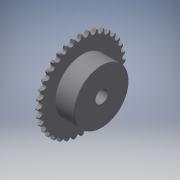
# Autodesk Inventor part: 22252-10380732036
Saved by Autodesk Inventor 2018 (Build 220112000, 112)
## iProperties
Category: PARTsolutions
Company: NORELEM
Created: 2018-08-05
Part Number: 22252-10380732036
Material: Generic
Catalog Web Link: www.cadenas.de
Description: 22252-Sprockets single 3/8“ x 7/32“ DIN ISO 606
Vendor: NORELEM
Document SubType Name: Modeling
Designer: psadmin
Manufacturer: NORELEM
Mass: 136.264 g
Surface Area: 270.64 cm^2
Volume: 136.264 cm^3
Density: 1 g/cm^3
Appearance: PSOLRGB-175-175-175
PSOL_IDENT_0: {$CADENAS_DATA\23d-libs\norelem\data\22000\22252.prj},174 {VTYP=3D},{NB=22252-10380732036},{LINA=222
PSOL_IDENT_1: 52-10380732036},{NN=22252},{DATE=25.07.2018 05:07:11},{GEOMDATE=17.06.2016 07:26:47},{VERSION=},{LIN
PSOL_IDENT_2: EID=430},{WBVAR=},{WBNUMERIC=}  {NB=22252-10380732036},{LINA=22252-10380732036},{KT=DUMMY},{BEST=222
PSOL_IDENT_3: 52-10380732036},{ISONR=06 B-1},{TZOLL=3/8\" x 7/32\"},{TMM=9,525 x 5,72},{ZZ=36},{D=113.0},{D1=109.2
PSOL_IDENT_4: 9},{D2=70},{D3=16},{B1=5.3},{L=30},{C=1},{R=10},{BS=Infotext},{INFO=Info},{FILTER=NORELEM,},{SAP=212
PSOL_IDENT_5: 278},{XC=1.300},{XD=6.350},{XF=1.800},{XG=0.000},{XH=0.000},{XI=0.000},{XJ=0.000},{XK=0.000},{XL=0.0
PSOL_IDENT_6: 00},{XM=0.000},{XN=0.000}
NN: 22252
NT: Sprockets single 3/8“ x 7/32“ DIN ISO 606
NB: 22252-10380732036
NBSYN: $BEST.
LINA: 22252-10380732036
BEST: 22252-10380732036
ISONR: 06 B-1
TZOLL: 3/8" x 7/32"
TMM: 9,525 x 5,72
ZZ: 36
D: 113
D1: 109.29
D2: 70
D3: 16
B1: 5.3
L: 30
C: 1
R: 10
BS: Infotext
INFO: Info
SUPPLIER: NORELEM
ARTICLENO: 22252-10380732036
BOMINFO: 22252-10380732036
CREATOR: CADENAS GmbH
Title: 22252-10380732036
Author: Cadenas PARTsolutions
Comments: Sprockets single 3/8“ x 7/32“ DIN ISO 606
Autodesk Inventor part; units mm, degrees
ref_plane "YZ Plane" through (0, 0, 0) normal (1, 0, 0) x (0, 1, 0)
ref_plane "XZ Plane" through (0, 0, 0) normal (0, 1, 0) x (-1, 0, 0)
ref_plane "XY Plane" through (0, 0, 0) normal (0, 0, 1) x (1, 0, 0)
sketch "Sketch_3" plane through (0, 0, 0) normal (1, 0, 0) x (0, 1, 0)
  arc A0 (0, 56.5) -> (-0.65, 56.4963) centre (0, 0) ccw
  line L0 (-0.65, 56.4963) -> (-1.7617, 53.3699)
  arc A1 (-4.485, 51.2642) -> (-1.7617, 53.3699) centre (-4.7626, 54.4371) ccw
  arc A2 (-7.5326, 52.8651) -> (-4.485, 51.2642) centre (-4.7626, 54.4371) ccw
  line L1 (-7.5326, 52.8651) -> (-9.1703, 55.7508)
  arc A3 (-9.1703, 55.7508) -> (-9.8111, 55.6416) centre (0, 0) ccw
  arc A4 (-9.8111, 55.6416) -> (-10.4506, 55.5251) centre (0, 0) ccw
  line L2 (-10.4506, 55.5251) -> (-11.0025, 52.2532)
  arc A5 (-13.3188, 49.7065) -> (-11.0025, 52.2532) centre (-14.1432, 52.783) ccw
  arc A6 (-16.5981, 50.7539) -> (-13.3188, 49.7065) centre (-14.1432, 52.783) ccw
  line L3 (-16.5981, 50.7539) -> (-18.7121, 53.3114)
  arc A7 (-18.7121, 53.3114) -> (-19.3241, 53.0926) centre (0, 0) ccw
  arc A8 (-19.3241, 53.0926) -> (-19.9337, 52.8668) centre (0, 0) ccw
  line L4 (-19.9337, 52.8668) -> (-19.9091, 49.5488)
  arc A9 (-21.7479, 46.6386) -> (-19.9091, 49.5488) centre (-23.094, 49.5252) ccw
  arc A10 (-25.1593, 47.1006) -> (-21.7479, 46.6386) centre (-23.094, 49.5252) ccw
  line L5 (-25.1593, 47.1006) -> (-27.6852, 49.2522)
  arc A11 (-27.6852, 49.2522) -> (-28.25, 48.9304) centre (0, 0) ccw
  arc A12 (-28.25, 48.9304) -> (-28.811, 48.6022) centre (0, 0) ccw
  line L6 (-28.811, 48.6022) -> (-28.2107, 45.3389)
  arc A13 (-29.5162, 42.1536) -> (-28.2107, 45.3389) centre (-31.3431, 44.7626) ccw
  arc A14 (-32.956, 42.0162) -> (-29.5162, 42.1536) centre (-31.3431, 44.7626) ccw
  line L7 (-32.956, 42.0162) -> (-35.8172, 43.6965)
  arc A15 (-35.8172, 43.6965) -> (-36.3175, 43.2815) centre (0, 0) ccw
  arc A16 (-36.3175, 43.2815) -> (-36.813, 42.8608) centre (0, 0) ccw
  line L8 (-36.813, 42.8608) -> (-35.6551, 39.7513)
  arc A17 (-36.3877, 36.3877) -> (-35.6551, 39.7513) centre (-38.6399, 38.6399) ccw
  arc A18 (-39.7513, 35.6551) -> (-36.3877, 36.3877) centre (-38.6399, 38.6399) ccw
  line L9 (-39.7513, 35.6551) -> (-42.8608, 36.813)
  arc A19 (-42.8608, 36.813) -> (-43.2815, 36.3175) centre (0, 0) ccw
  arc A20 (-43.2815, 36.3175) -> (-43.6965, 35.8172) centre (0, 0) ccw
  line L10 (-43.6965, 35.8172) -> (-42.0162, 32.956)
  arc A21 (-42.1536, 29.5162) -> (-42.0162, 32.956) centre (-44.7626, 31.3431) ccw
  arc A22 (-45.3389, 28.2107) -> (-42.1536, 29.5162) centre (-44.7626, 31.3431) ccw
  line L11 (-45.3389, 28.2107) -> (-48.6022, 28.811)
  arc A23 (-48.6022, 28.811) -> (-48.9304, 28.25) centre (0, 0) ccw
  arc A24 (-48.9304, 28.25) -> (-49.2522, 27.6852) centre (0, 0) ccw
  line L12 (-49.2522, 27.6852) -> (-47.1006, 25.1593)
  arc A25 (-46.6386, 21.7479) -> (-47.1006, 25.1593) centre (-49.5252, 23.094) ccw
  arc A26 (-49.5488, 19.9091) -> (-46.6386, 21.7479) centre (-49.5252, 23.094) ccw
  line L13 (-49.5488, 19.9091) -> (-52.8668, 19.9337)
  arc A27 (-52.8668, 19.9337) -> (-53.0926, 19.3241) centre (0, 0) ccw
  arc A28 (-53.0926, 19.3241) -> (-53.3114, 18.7121) centre (0, 0) ccw
  line L14 (-53.3114, 18.7121) -> (-50.7539, 16.5981)
  arc A29 (-49.7065, 13.3188) -> (-50.7539, 16.5981) centre (-52.783, 14.1432) ccw
  arc A30 (-52.2532, 11.0025) -> (-49.7065, 13.3188) centre (-52.783, 14.1432) ccw
  line L15 (-52.2532, 11.0025) -> (-55.5251, 10.4506)
  arc A31 (-55.5251, 10.4506) -> (-55.6416, 9.8111) centre (0, 0) ccw
  arc A32 (-55.6416, 9.8111) -> (-55.7508, 9.1703) centre (0, 0) ccw
  line L16 (-55.7508, 9.1703) -> (-52.8651, 7.5326)
  arc A33 (-51.2642, 4.485) -> (-52.8651, 7.5326) centre (-54.4371, 4.7626) ccw
  arc A34 (-53.3699, 1.7617) -> (-51.2642, 4.485) centre (-54.4371, 4.7626) ccw
  line L17 (-53.3699, 1.7617) -> (-56.4963, 0.65)
  arc A35 (-56.4963, 0.65) -> (-56.5, 0) centre (0, 0) ccw
  arc A36 (-56.5, 0) -> (-56.4963, -0.65) centre (0, 0) ccw
  line L18 (-56.4963, -0.65) -> (-53.3699, -1.7617)
  arc A37 (-51.2642, -4.485) -> (-53.3699, -1.7617) centre (-54.4371, -4.7626) ccw
  arc A38 (-52.8651, -7.5326) -> (-51.2642, -4.485) centre (-54.4371, -4.7626) ccw
  line L19 (-52.8651, -7.5326) -> (-55.7508, -9.1703)
  arc A39 (-55.7508, -9.1703) -> (-55.6416, -9.8111) centre (0, 0) ccw
  arc A40 (-55.6416, -9.8111) -> (-55.5251, -10.4506) centre (0, 0) ccw
  line L20 (-55.5251, -10.4506) -> (-52.2532, -11.0025)
  arc A41 (-49.7065, -13.3188) -> (-52.2532, -11.0025) centre (-52.783, -14.1432) ccw
  arc A42 (-50.7539, -16.5981) -> (-49.7065, -13.3188) centre (-52.783, -14.1432) ccw
  line L21 (-50.7539, -16.5981) -> (-53.3114, -18.7121)
  arc A43 (-53.3114, -18.7121) -> (-53.0926, -19.3241) centre (0, 0) ccw
  arc A44 (-53.0926, -19.3241) -> (-52.8668, -19.9337) centre (0, 0) ccw
  line L22 (-52.8668, -19.9337) -> (-49.5488, -19.9091)
  arc A45 (-46.6386, -21.7479) -> (-49.5488, -19.9091) centre (-49.5252, -23.094) ccw
  arc A46 (-47.1006, -25.1593) -> (-46.6386, -21.7479) centre (-49.5252, -23.094) ccw
  line L23 (-47.1006, -25.1593) -> (-49.2522, -27.6852)
  arc A47 (-49.2522, -27.6852) -> (-48.9304, -28.25) centre (0, 0) ccw
  arc A48 (-48.9304, -28.25) -> (-48.6022, -28.811) centre (0, 0) ccw
  line L24 (-48.6022, -28.811) -> (-45.3389, -28.2107)
  arc A49 (-42.1536, -29.5162) -> (-45.3389, -28.2107) centre (-44.7626, -31.3431) ccw
  arc A50 (-42.0162, -32.956) -> (-42.1536, -29.5162) centre (-44.7626, -31.3431) ccw
  line L25 (-42.0162, -32.956) -> (-43.6965, -35.8172)
  arc A51 (-43.6965, -35.8172) -> (-43.2815, -36.3175) centre (0, 0) ccw
  arc A52 (-43.2815, -36.3175) -> (-42.8608, -36.813) centre (0, 0) ccw
  line L26 (-42.8608, -36.813) -> (-39.7513, -35.6551)
  arc A53 (-36.3877, -36.3877) -> (-39.7513, -35.6551) centre (-38.6399, -38.6399) ccw
  arc A54 (-35.6551, -39.7513) -> (-36.3877, -36.3877) centre (-38.6399, -38.6399) ccw
  line L27 (-35.6551, -39.7513) -> (-36.813, -42.8608)
  arc A55 (-36.813, -42.8608) -> (-36.3175, -43.2815) centre (0, 0) ccw
  arc A56 (-36.3175, -43.2815) -> (-35.8172, -43.6965) centre (0, 0) ccw
  line L28 (-35.8172, -43.6965) -> (-32.956, -42.0162)
  arc A57 (-29.5162, -42.1536) -> (-32.956, -42.0162) centre (-31.3431, -44.7626) ccw
  arc A58 (-28.2107, -45.3389) -> (-29.5162, -42.1536) centre (-31.3431, -44.7626) ccw
  line L29 (-28.2107, -45.3389) -> (-28.811, -48.6022)
  arc A59 (-28.811, -48.6022) -> (-28.25, -48.9304) centre (0, 0) ccw
  arc A60 (-28.25, -48.9304) -> (-27.6852, -49.2522) centre (0, 0) ccw
  line L30 (-27.6852, -49.2522) -> (-25.1593, -47.1006)
  arc A61 (-21.7479, -46.6386) -> (-25.1593, -47.1006) centre (-23.094, -49.5252) ccw
  arc A62 (-19.9091, -49.5488) -> (-21.7479, -46.6386) centre (-23.094, -49.5252) ccw
  line L31 (-19.9091, -49.5488) -> (-19.9337, -52.8668)
  arc A63 (-19.9337, -52.8668) -> (-19.3241, -53.0926) centre (0, 0) ccw
  arc A64 (-19.3241, -53.0926) -> (-18.7121, -53.3114) centre (0, 0) ccw
  line L32 (-18.7121, -53.3114) -> (-16.5981, -50.7539)
  arc A65 (-13.3188, -49.7065) -> (-16.5981, -50.7539) centre (-14.1432, -52.783) ccw
  arc A66 (-11.0025, -52.2532) -> (-13.3188, -49.7065) centre (-14.1432, -52.783) ccw
  line L33 (-11.0025, -52.2532) -> (-10.4506, -55.5251)
  arc A67 (-10.4506, -55.5251) -> (-9.8111, -55.6416) centre (0, 0) ccw
  arc A68 (-9.8111, -55.6416) -> (-9.1703, -55.7508) centre (0, 0) ccw
  line L34 (-9.1703, -55.7508) -> (-7.5326, -52.8651)
  arc A69 (-4.485, -51.2642) -> (-7.5326, -52.8651) centre (-4.7626, -54.4371) ccw
  arc A70 (-1.7617, -53.3699) -> (-4.485, -51.2642) centre (-4.7626, -54.4371) ccw
  line L35 (-1.7617, -53.3699) -> (-0.65, -56.4963)
  arc A71 (-0.65, -56.4963) -> (0, -56.5) centre (0, 0) ccw
  arc A72 (0, -56.5) -> (0.65, -56.4963) centre (0, 0) ccw
  line L36 (0.65, -56.4963) -> (1.7617, -53.3699)
  arc A73 (4.485, -51.2642) -> (1.7617, -53.3699) centre (4.7626, -54.4371) ccw
  arc A74 (7.5326, -52.8651) -> (4.485, -51.2642) centre (4.7626, -54.4371) ccw
  line L37 (7.5326, -52.8651) -> (9.1703, -55.7508)
  arc A75 (9.1703, -55.7508) -> (9.8111, -55.6416) centre (0, 0) ccw
  arc A76 (9.8111, -55.6416) -> (10.4506, -55.5251) centre (0, 0) ccw
  line L38 (10.4506, -55.5251) -> (11.0025, -52.2532)
  arc A77 (13.3188, -49.7065) -> (11.0025, -52.2532) centre (14.1432, -52.783) ccw
  arc A78 (16.5981, -50.7539) -> (13.3188, -49.7065) centre (14.1432, -52.783) ccw
  line L39 (16.5981, -50.7539) -> (18.7121, -53.3114)
  arc A79 (18.7121, -53.3114) -> (19.3241, -53.0926) centre (0, 0) ccw
  arc A80 (19.3241, -53.0926) -> (19.9337, -52.8668) centre (0, 0) ccw
  line L40 (19.9337, -52.8668) -> (19.9091, -49.5488)
  arc A81 (21.7479, -46.6386) -> (19.9091, -49.5488) centre (23.094, -49.5252) ccw
  arc A82 (25.1593, -47.1006) -> (21.7479, -46.6386) centre (23.094, -49.5252) ccw
  line L41 (25.1593, -47.1006) -> (27.6852, -49.2522)
  arc A83 (27.6852, -49.2522) -> (28.25, -48.9304) centre (0, 0) ccw
  arc A84 (28.25, -48.9304) -> (28.811, -48.6022) centre (0, 0) ccw
  line L42 (28.811, -48.6022) -> (28.2107, -45.3389)
  arc A85 (29.5162, -42.1536) -> (28.2107, -45.3389) centre (31.3431, -44.7626) ccw
  arc A86 (32.956, -42.0162) -> (29.5162, -42.1536) centre (31.3431, -44.7626) ccw
  line L43 (32.956, -42.0162) -> (35.8172, -43.6965)
  arc A87 (35.8172, -43.6965) -> (36.3175, -43.2815) centre (0, 0) ccw
  arc A88 (36.3175, -43.2815) -> (36.813, -42.8608) centre (0, 0) ccw
  line L44 (36.813, -42.8608) -> (35.6551, -39.7513)
  arc A89 (36.3877, -36.3877) -> (35.6551, -39.7513) centre (38.6399, -38.6399) ccw
  arc A90 (39.7513, -35.6551) -> (36.3877, -36.3877) centre (38.6399, -38.6399) ccw
  line L45 (39.7513, -35.6551) -> (42.8608, -36.813)
  arc A91 (42.8608, -36.813) -> (43.2815, -36.3175) centre (0, 0) ccw
  arc A92 (43.2815, -36.3175) -> (43.6965, -35.8172) centre (0, 0) ccw
  line L46 (43.6965, -35.8172) -> (42.0162, -32.956)
  arc A93 (42.1536, -29.5162) -> (42.0162, -32.956) centre (44.7626, -31.3431) ccw
  arc A94 (45.3389, -28.2107) -> (42.1536, -29.5162) centre (44.7626, -31.3431) ccw
  line L47 (45.3389, -28.2107) -> (48.6022, -28.811)
  arc A95 (48.6022, -28.811) -> (48.9304, -28.25) centre (0, 0) ccw
  arc A96 (48.9304, -28.25) -> (49.2522, -27.6852) centre (0, 0) ccw
  line L48 (49.2522, -27.6852) -> (47.1006, -25.1593)
  arc A97 (46.6386, -21.7479) -> (47.1006, -25.1593) centre (49.5252, -23.094) ccw
  arc A98 (49.5488, -19.9091) -> (46.6386, -21.7479) centre (49.5252, -23.094) ccw
  line L49 (49.5488, -19.9091) -> (52.8668, -19.9337)
  arc A99 (52.8668, -19.9337) -> (53.0926, -19.3241) centre (0, 0) ccw
  arc A100 (53.0926, -19.3241) -> (53.3114, -18.7121) centre (0, 0) ccw
  line L50 (53.3114, -18.7121) -> (50.7539, -16.5981)
  arc A101 (49.7065, -13.3188) -> (50.7539, -16.5981) centre (52.783, -14.1432) ccw
  arc A102 (52.2532, -11.0025) -> (49.7065, -13.3188) centre (52.783, -14.1432) ccw
  line L51 (52.2532, -11.0025) -> (55.5251, -10.4506)
  arc A103 (55.5251, -10.4506) -> (55.6416, -9.8111) centre (0, 0) ccw
  arc A104 (55.6416, -9.8111) -> (55.7508, -9.1703) centre (0, 0) ccw
  line L52 (55.7508, -9.1703) -> (52.8651, -7.5326)
  arc A105 (51.2642, -4.485) -> (52.8651, -7.5326) centre (54.4371, -4.7626) ccw
  arc A106 (53.3699, -1.7617) -> (51.2642, -4.485) centre (54.4371, -4.7626) ccw
  line L53 (53.3699, -1.7617) -> (56.4963, -0.65)
  arc A107 (56.4963, -0.65) -> (56.5, 0) centre (0, 0) ccw
  arc A108 (56.5, 0) -> (56.4963, 0.65) centre (0, 0) ccw
  line L54 (56.4963, 0.65) -> (53.3699, 1.7617)
  arc A109 (51.2642, 4.485) -> (53.3699, 1.7617) centre (54.4371, 4.7626) ccw
  arc A110 (52.8651, 7.5326) -> (51.2642, 4.485) centre (54.4371, 4.7626) ccw
  line L55 (52.8651, 7.5326) -> (55.7508, 9.1703)
  arc A111 (55.7508, 9.1703) -> (55.6416, 9.8111) centre (0, 0) ccw
  arc A112 (55.6416, 9.8111) -> (55.5251, 10.4506) centre (0, 0) ccw
  line L56 (55.5251, 10.4506) -> (52.2532, 11.0025)
  arc A113 (49.7065, 13.3188) -> (52.2532, 11.0025) centre (52.783, 14.1432) ccw
  arc A114 (50.7539, 16.5981) -> (49.7065, 13.3188) centre (52.783, 14.1432) ccw
  line L57 (50.7539, 16.5981) -> (53.3114, 18.7121)
  arc A115 (53.3114, 18.7121) -> (53.0926, 19.3241) centre (0, 0) ccw
  arc A116 (53.0926, 19.3241) -> (52.8668, 19.9337) centre (0, 0) ccw
  line L58 (52.8668, 19.9337) -> (49.5488, 19.9091)
  arc A117 (46.6386, 21.7479) -> (49.5488, 19.9091) centre (49.5252, 23.094) ccw
  arc A118 (47.1006, 25.1593) -> (46.6386, 21.7479) centre (49.5252, 23.094) ccw
  line L59 (47.1006, 25.1593) -> (49.2522, 27.6852)
  arc A119 (49.2522, 27.6852) -> (48.9304, 28.25) centre (0, 0) ccw
  arc A120 (48.9304, 28.25) -> (48.6022, 28.811) centre (0, 0) ccw
  line L60 (48.6022, 28.811) -> (45.3389, 28.2107)
  arc A121 (42.1536, 29.5162) -> (45.3389, 28.2107) centre (44.7626, 31.3431) ccw
  arc A122 (42.0162, 32.956) -> (42.1536, 29.5162) centre (44.7626, 31.3431) ccw
  line L61 (42.0162, 32.956) -> (43.6965, 35.8172)
  arc A123 (43.6965, 35.8172) -> (43.2815, 36.3175) centre (0, 0) ccw
  arc A124 (43.2815, 36.3175) -> (42.8608, 36.813) centre (0, 0) ccw
  line L62 (42.8608, 36.813) -> (39.7513, 35.6551)
  arc A125 (36.3877, 36.3877) -> (39.7513, 35.6551) centre (38.6399, 38.6399) ccw
  arc A126 (35.6551, 39.7513) -> (36.3877, 36.3877) centre (38.6399, 38.6399) ccw
  line L63 (35.6551, 39.7513) -> (36.813, 42.8608)
  arc A127 (36.813, 42.8608) -> (36.3175, 43.2815) centre (0, 0) ccw
  arc A128 (36.3175, 43.2815) -> (35.8172, 43.6965) centre (0, 0) ccw
  line L64 (35.8172, 43.6965) -> (32.956, 42.0162)
  arc A129 (29.5162, 42.1536) -> (32.956, 42.0162) centre (31.3431, 44.7626) ccw
  arc A130 (28.2107, 45.3389) -> (29.5162, 42.1536) centre (31.3431, 44.7626) ccw
  line L65 (28.2107, 45.3389) -> (28.811, 48.6022)
  arc A131 (28.811, 48.6022) -> (28.25, 48.9304) centre (0, 0) ccw
  arc A132 (28.25, 48.9304) -> (27.6852, 49.2522) centre (0, 0) ccw
  line L66 (27.6852, 49.2522) -> (25.1593, 47.1006)
  arc A133 (21.7479, 46.6386) -> (25.1593, 47.1006) centre (23.094, 49.5252) ccw
  arc A134 (19.9091, 49.5488) -> (21.7479, 46.6386) centre (23.094, 49.5252) ccw
  line L67 (19.9091, 49.5488) -> (19.9337, 52.8668)
  arc A135 (19.9337, 52.8668) -> (19.3241, 53.0926) centre (0, 0) ccw
  arc A136 (19.3241, 53.0926) -> (18.7121, 53.3114) centre (0, 0) ccw
  line L68 (18.7121, 53.3114) -> (16.5981, 50.7539)
  arc A137 (13.3188, 49.7065) -> (16.5981, 50.7539) centre (14.1432, 52.783) ccw
  arc A138 (11.0025, 52.2532) -> (13.3188, 49.7065) centre (14.1432, 52.783) ccw
  line L69 (11.0025, 52.2532) -> (10.4506, 55.5251)
  arc A139 (10.4506, 55.5251) -> (9.8111, 55.6416) centre (0, 0) ccw
  arc A140 (9.8111, 55.6416) -> (9.1703, 55.7508) centre (0, 0) ccw
  line L70 (9.1703, 55.7508) -> (7.5326, 52.8651)
  arc A141 (4.485, 51.2642) -> (7.5326, 52.8651) centre (4.7626, 54.4371) ccw
  arc A142 (1.7617, 53.3699) -> (4.485, 51.2642) centre (4.7626, 54.4371) ccw
  line L71 (1.7617, 53.3699) -> (0.65, 56.4963)
  arc A143 (0.65, 56.4963) -> (0, 56.5) centre (0, 0) ccw
  circle A144 centre (0, 0) radius 8
  constraints: 288 point on circle, 145 centre point, 144 end point
extrude "Extrusion1" add sketch "Sketch_3" along normal blind 30
sketch "Sketch_5" plane through (0, 0, 0) normal (0, 0, 1) x (1, 0, 0)
  line L0 (30, 0) -> (-2.65, 0)
  line L1 (-2.65, 61.5) -> (-2.65, 54.7)
  line L2 (-2.65, 54.7) -> (0, 54.7)
  arc A0 (1, 56.5) -> (0, 54.7) centre (9.1951, 50.7694) ccw
  line L3 (1, 56.5) -> (4.3, 56.5)
  arc A1 (5.3, 54.7) -> (4.3, 56.5) centre (-3.8951, 50.7694) ccw
  line L4 (5.3, 54.7) -> (5.3, 35)
  line L5 (5.3, 35) -> (29.5, 35)
  line L6 (29.5, 35) -> (30, 34.5)
  line L7 (30, 34.5) -> (30, 61.5)
  line L8 (30, 61.5) -> (-2.65, 61.5)
  constraints: 18 end point, 4 point on circle, 2 centre point
revolve "Revolution1" cut sketch "Sketch_5" angle 360 about axis through (30, 0, 0) along (1, 0, 0)
body "Solid1"
